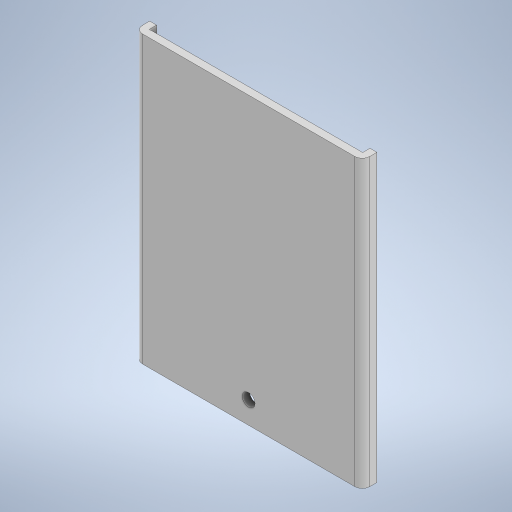
# Autodesk Inventor part: 커튼 정면 커버
Saved by Autodesk Inventor 2023.1 (Build 271208000, 208)
## iProperties
Created: 2022-09-03
Part Number: 커튼 정면 커버
Material: 일반
Document SubType Name: Modeling
Designer: fly01
Density: 1 g/cm^3
Appearance: 기본값
Author: fly01
Autodesk Inventor part; units mm, degrees
ref_plane "YZ Plane" through (0, 0, 0) normal (1, 0, 0) x (0, 1, 0)
ref_plane "XZ Plane" through (0, 0, 0) normal (0, 1, 0) x (-1, 0, 0)
ref_plane "XY Plane" through (0, 0, 0) normal (0, 0, 1) x (1, 0, 0)
sketch "스케치1" plane through (0, 0, 0) normal (0, 0, 1) x (1, 0, 0)
  line L0 (-31, -39) -> (31, -39)
  line L1 (31, -39) -> (31, 39)
  line L2 (31, 39) -> (-31, 39)
  line L3 (-31, 39) -> (-31, -39)
  line L4 (-31, -39) -> (31, 39) construction
  line L5 (31, -39) -> (-31, 39) construction
  line L6 (-29.1, 37.1) -> (29.1, 37.1)
  line L7 (29.1, 37.1) -> (29.1, -37.1)
  line L8 (29.1, -37.1) -> (-29.1, -37.1)
  line L9 (-29.1, -37.1) -> (-29.1, 37.1)
  line L10 (-29.1, 37.1) -> (-29.1, 39)
  line L11 (29.1, 37.1) -> (29.1, 39)
  point P0 (0, 0)
  dimension "d0" = 62
  dimension "d1" = 78
  dimension "d2" = 1.9
  constraints: 24 end point, 4 parallel, 4 perpendicular, 2 midpoint, 2 point on line, 1 horizontal, 3 other
  measures "d0" distance of L1.end L2.end
  measures "d1" distance of L0.end L1.end
  measures "d2" distance between parallel lines of L2 L6
extrude "돌출1" add sketch "스케치1" against normal blind 2 contours L3 L2 L10 L9 L8 L7 L11 L1 L0
extrude "돌출2" add sketch "스케치1" along normal blind 2
sketch "스케치2" plane through (0, 0, 0) normal (0, 0, -1) x (-1, 0, 0)
  line L0 (-3, -45) -> (3, -45)
  line L1 (3, -45) -> (3, -33)
  line L2 (3, -33) -> (-3, -33) construction
  line L3 (-3, -33) -> (-3, -45)
  line L4 (31, -39) -> (-31, -39) projected
  line L5 (-3, -45) -> (3, -33) construction
  line L6 (3, -45) -> (-3, -33) construction
  circle A0 centre (0, -33) radius 3
  circle A1 centre (0, -33) radius 1.75
  point P0 (0, 0)
  point P1 (0, -39)
  point P2 (-3, -39)
  point P3 (3, -39)
  dimension "d7" = 12
  dimension "d8" = 6
  dimension "d9" = 3.5
  constraints: 12 end point, 4 midpoint, 2 parallel, 1 centre point, 1 coincident, 1 horizontal, 1 perpendicular, 3 other
  measures "d7" distance of L0.end L1.end
  measures "d8" distance of L1.end L2.end
  measures "d9" diameter of A1
extrude "돌출4" cut sketch "스케치2" against normal blind 2 contours A1
fillet "모깎기1" radius 2 2 edges at (-31, 0, 2) (31, 0, 2)
